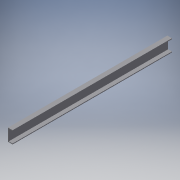
# Autodesk Inventor part: NASA-20-OP-01
Saved by Autodesk Inventor 2019 (Build 230136000, 136)
## iProperties
Created: 2019-09-07
Part Number: NASA-20-OP-01
Material: Generic
Document SubType Name: Modeling
Designer: Rick Szalay
Density: 1 g/cm^3
Appearance: Default
Author: Rick Szalay
Autodesk Inventor part; units mm, degrees
ref_plane "YZ Plane" through (0, 0, 0) normal (1, 0, 0) x (0, 1, 0)
ref_plane "XZ Plane" through (0, 0, 0) normal (0, 1, 0) x (-1, 0, 0)
ref_plane "XY Plane" through (0, 0, 0) normal (0, 0, 1) x (1, 0, 0)
sketch "Sketch1" plane through (0, 0, 0) normal (0, 0, 1) x (1, 0, 0)
  line L0 (0, 25.4) -> (0, -25.4)
  line L1 (0, -25.4) -> (19.05, -25.4)
  line L2 (0, 25.4) -> (19.05, 25.4)
  line L3 (19.05, 25.4) -> (19.05, 22.225)
  line L4 (19.05, 22.225) -> (3.048, 22.225)
  line L5 (3.048, 22.225) -> (3.048, -22.225)
  line L6 (3.048, -22.225) -> (19.05, -22.225)
  line L7 (19.05, -22.225) -> (19.05, -25.4)
  point P0 (0, 0)
  point P1 (0, 0)
  dimension "d0" = 50.8
  dimension "d1" = 19.05
  dimension "d2" = 3.175
  dimension "d3" = 16.002
  constraints: 16 end point, 5 perpendicular, 2 equal length, 2 vertical, 1 coincident, 1 horizontal, 1 midpoint, 1 point on line
  measures "d0" distance of L0.start L0.end
  measures "d1" distance of L0.start L2.end
  measures "d2" distance between parallel lines of L4 L2
  measures "d3" distance between parallel lines of L5 L7
extrude "Extrusion1" add sketch "Sketch1" along normal mid plane 660.4
fillet "Fillet1" radius 1.5875 4 edges at (3.048, 22.225, 0) (3.048, -22.225, 0) (19.05, -22.225, 0) (19.05, 22.225, 0)
sketch "Sketch2" plane through (3.048, -20.6375, -330.2) normal (1, 0, 0) x (0, 0, -1)
  point P0 (-330.2, 20.6375)
  point P1 (-177.8, 20.6375)
  point P2 (-482.6, 20.6375)
  dimension "d7" = 304.8
  dimension "d8" = 152.4
  constraints: 2 horizontal alignment
  measures "d7" distance of point (-482.6, 20.637) point (-177.8, 20.637)
  measures "d8" distance of point (-177.8, 20.637) point (-330.2, 20.637)
hole "Hole1" at (3.048, 0, -152.4) at (3.048, 0, 152.4) direction (-1, 0, 0) diameter 6.35 depth 25.4 tip angle 118
equation "\"d4\" = Length"
equation "\"Length\" = 660.4"
body "Solid1"
